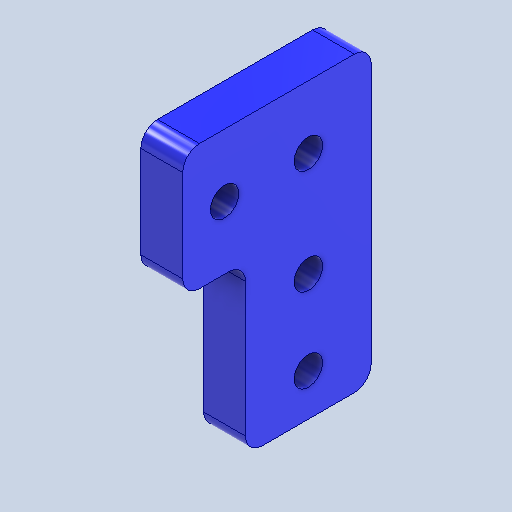
# Autodesk Inventor part: ball_loading_v1_Plate_ASP_F_3
Saved by Autodesk Inventor 2025.1 (Build 291241000, 241)
## iProperties
Created: 2024-11-12
Part Number: ball_loading_v1_Plate_ASP_F_3
Material: ABS プラスチック
Document SubType Name: Modeling
Designer: haruy
Density: 1.06 g/cm^3
Appearance: 青 - 壁塗料 - 光沢
Author: haruy
Autodesk Inventor part; units mm, degrees
ref_plane "YZ Plane" through (0, 0, 0) normal (1, 0, 0) x (0, 1, 0)
ref_plane "XZ Plane" through (0, 0, 0) normal (0, 1, 0) x (-1, 0, 0)
ref_plane "XY Plane" through (0, 0, 0) normal (0, 0, 1) x (1, 0, 0)
sketch "スケッチ1" plane through (0, 0, 0) normal (1, 0, 0) x (0, 1, 0)
  line L0 (-144.8102, -220.9081) -> (-144.8102, 234.0919)
  line L1 (-144.8102, -220.9081) -> (145.1898, -220.9081)
  line L2 (145.1898, -220.9081) -> (145.1898, -205.9081)
  line L3 (145.1898, -205.9081) -> (-144.8102, -205.9081)
  line L4 (-144.8102, -205.9081) -> (-144.8102, -220.9081)
  line L5 (145.1898, 234.0919) -> (145.1898, -220.9081)
  line L6 (145.1898, -220.9081) -> (160.1898, -220.9081)
  line L7 (160.1898, 234.0919) -> (160.1898, -220.9081)
  line L8 (0.1898, -205.9081) -> (0.1898, -220.9081)
  line L9 (125.1898, -205.9081) -> (125.1898, -220.9081)
  line L10 (145.1898, -198.4081) -> (160.1898, -198.4081)
  circle A0 centre (130.1898, -213.4081) radius 1.7
  circle A1 centre (140.1898, -213.4081) radius 1.7
  circle A2 centre (152.6898, -213.4081) radius 1.7
  circle A3 centre (152.6898, -203.4081) radius 1.7
  point P0 (0, 0)
  point P1 (-54.8102, -185.9081)
  point P2 (-152.3102, -203.4081)
  point P3 (-152.3102, -213.4081)
  point P4 (-139.8102, -213.4081)
  point P5 (-129.8102, -213.4081)
  dimension "d0" = 15
  dimension "d1" = 0
  dimension "d2" = 10
  dimension "d3" = 7.5
  dimension "d4" = 10
  dimension "d5" = 5
  dimension "d6" = 7.5
  dimension "d7" = 7.5
  dimension "d8" = 7.5
  dimension "d9" = 7.5
  dimension "d10" = 5
  dimension "d11" = 5
  dimension "d12" = 3.4
  dimension "d13" = 3.4
  dimension "d14" = 3.4
  dimension "d15" = 3.4
  constraints: 22 end point, 4 centre point, 4 coincident, 4 point on line, 4 symmetric about line, 3 perpendicular, 2 midpoint, 2 parallel, 1 horizontal
  measures "d0" distance of L2.end L1.end
  measures "d1" distance between parallel lines of L5 L2
  measures "d2" distance of point (152.69, -213.408) point (152.69, -203.408)
  measures "d3" distance from line of L3 point (140.19, -213.408)
  measures "d4" distance of point (130.19, -213.408) point (140.19, -213.408)
  measures "d5" distance from line of point (140.19, -213.408) L2
  measures "d6" distance from line of L1 point (130.19, -213.408)
  measures "d7" distance from line of point (152.69, -213.408) L6
  measures "d8" distance from line of L7 point (152.69, -213.408)
  measures "d9" distance from line of L7 point (152.69, -203.408)
  measures "d10" distance from line of L9 point (130.19, -213.408)
  measures "d11" distance from line of L10 point (152.69, -203.408)
  measures "d12" diameter of A0
  measures "d13" diameter of A1
  measures "d14" diameter of A2
  measures "d15" diameter of A3
extrude "押し出し1" add sketch "スケッチ1" along normal blind 5 contours L9 L3 L2 L1 | L2 L5 L10 L7 L6
fillet "フィレット1" radius 2 6 edges at (2.5, 160.1898, -220.9081) (2.5, 160.1898, -198.4081) (2.5, 145.1898, -198.4081) (2.5, 145.1898, -205.9081) (2.5, 125.1898, -205.9081) (2.5, 125.1898, -220.9081)
equation "\"d6\" = d3"
equation "\"d9\" = d8"
